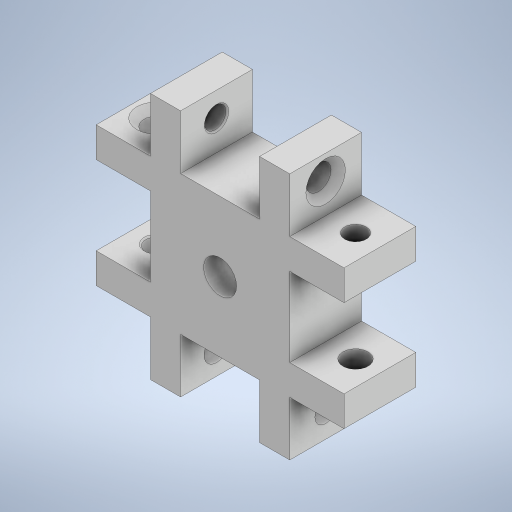
# Autodesk Inventor part: GripperMotorHinges
Saved by Autodesk Inventor 2023 (Build 270158000, 158)
## iProperties
Created: 2023-06-03
Part Number: GripperMotorHinges
Material: Ogólny
Document SubType Name: Modeling
Designer: Kamil
Density: 1 g/cm^3
Appearance: Domyślna
Author: Kamil
Autodesk Inventor part; units mm, degrees
ref_plane "YZ Plane" through (0, 0, 0) normal (1, 0, 0) x (0, 1, 0)
ref_plane "XZ Plane" through (0, 0, 0) normal (0, 1, 0) x (-1, 0, 0)
ref_plane "XY Plane" through (0, 0, 0) normal (0, 0, 1) x (1, 0, 0)
sketch "Szkic1" plane through (0, 0, 0) normal (0, 0, 1) x (1, 0, 0)
  line L0 (0, -7.56) -> (0, 0)
  line L1 (0, 19.4) -> (0, 26.96)
  line L2 (-4.2, 4.2) -> (-11.76, 4.2)
  line L3 (-11.76, 15.2) -> (-4.2, 15.2)
  line L4 (15.2, 15.2) -> (22.76, 15.2)
  line L5 (15.2, 4.2) -> (22.76, 4.2)
  line L6 (-4.2, 26.96) -> (-4.2, 19.4)
  line L7 (-4.2, 19.4) -> (-11.76, 19.4)
  line L8 (-4.2, 15.2) -> (-4.2, 4.2)
  line L9 (-4.2, 0) -> (-4.2, -7.56)
  line L10 (-11.76, 0) -> (-4.2, 0)
  line L11 (15.2, -7.56) -> (11, -7.56)
  line L12 (0, -7.56) -> (-4.2, -7.56)
  line L13 (0, 0) -> (11, 0)
  line L14 (15.2, 0) -> (22.76, 0)
  line L15 (11, 26.96) -> (11, 19.4)
  line L16 (11, 0) -> (11, -7.56)
  line L17 (15.2, -7.56) -> (15.2, 0)
  line L18 (15.2, 4.2) -> (15.2, 15.2)
  line L19 (15.2, 19.4) -> (15.2, 26.96)
  line L20 (22.76, 19.4) -> (15.2, 19.4)
  line L21 (11, 19.4) -> (0, 19.4)
  line L22 (22.76, 19.4) -> (22.76, 15.2)
  line L23 (22.76, 4.2) -> (22.76, 0)
  line L24 (-4.2, 26.96) -> (0, 26.96)
  line L25 (11, 26.96) -> (15.2, 26.96)
  line L26 (-11.76, 0) -> (-11.76, 4.2)
  line L27 (-11.76, 15.2) -> (-11.76, 19.4)
  circle A0 centre (5.5, 9.7) radius 2.3
  dimension "d0" = 4.6
  constraints: 56 end point, 8 parallel, 8 perpendicular, 2 horizontal, 1 centre point, 1 coincident
  measures "d0" diameter of A0
extrude "Wyciągnięcie proste1" add sketch "Szkic1" along normal blind 10
sketch "Szkic2" plane through (-11.76, 19.4, 0) normal (0, 1, 0) x (1, 0, 0)
  line L0 (7.56, 0) -> (0, 0) projected
  line L1 (0, 0) -> (0, -10) projected
  line L2 (7.56, -10) -> (0, -10) projected
  line L3 (7.56, 0) -> (7.56, -10) projected
  line L4 (34.52, 0) -> (26.96, 0) projected
  line L5 (26.96, 0) -> (26.96, -10) projected
  line L6 (34.52, -10) -> (26.96, -10) projected
  line L7 (34.52, 0) -> (34.52, -10) projected
  line L8 (0, 0) -> (0, -10) projected
  line L9 (0, -5) -> (3.4, -5)
  line L10 (34.52, 0) -> (34.52, -10) projected
  line L11 (34.52, -5) -> (31.12, -5)
  circle A0 centre (3.4, -5) radius 1.75
  circle A1 centre (31.12, -5) radius 1.75
  point P0 (11.76, 0)
  dimension "d3" = 3.4
  dimension "d4" = 3.4
  dimension "d5" = 3.5
  dimension "d6" = 3.5
  constraints: 4 end point, 2 centre point, 2 coincident, 2 horizontal, 2 midpoint
  measures "d3" distance of L9.start L9.end
  measures "d4" distance of L11.start L11.end
  measures "d5" diameter of A0
  measures "d6" diameter of A1
extrude "Wyciągnięcie proste2" cut sketch "Szkic2" against normal through all contours A0 | A1
sketch "Szkic3" plane through (-4.2, -7.56, 0) normal (-1, 0, 0) x (0, 0, 1)
  line L0 (0, 7.56) -> (0, 0) projected
  line L1 (0, 0) -> (10, 0) projected
  line L2 (10, 7.56) -> (10, 0) projected
  line L3 (0, 7.56) -> (10, 7.56) projected
  line L4 (0, 34.52) -> (0, 26.96) projected
  line L5 (0, 26.96) -> (10, 26.96) projected
  line L6 (10, 34.52) -> (10, 26.96) projected
  line L7 (0, 34.52) -> (10, 34.52) projected
  line L8 (5, 0) -> (5, 3.4)
  line L9 (0, 34.52) -> (10, 34.52) projected
  line L10 (5, 34.52) -> (5, 31.12)
  circle A0 centre (5, 3.4) radius 1.75
  circle A1 centre (5, 31.12) radius 1.75
  point P0 (0, 7.56)
  dimension "d9" = 3.4
  dimension "d10" = 3.4
  dimension "d11" = 3.5
  dimension "d12" = 3.5
  constraints: 4 end point, 2 centre point, 2 coincident, 2 midpoint, 2 vertical
  measures "d9" distance of L8.start L8.end
  measures "d10" distance of L10.start L10.end
  measures "d11" diameter of A0
  measures "d12" diameter of A1
extrude "Wyciągnięcie proste3" cut sketch "Szkic3" against normal through all contours A0 | A1
chamfer "Faza2" distance 1 angle 45 4 edges at (-4.2, -4.16, 3.25) (17.61, 0, 5) (15.2, 23.56, 3.25) (-10.11, 19.4, 5)
sketch "Szkic8" plane through (15.2, -7.56, 0) normal (1, 0, 0) x (0, 0, -1)
  circle A0 centre (-5, 3.4) radius 1.75 projected
  circle A1 centre (-5, 3.4) radius 1.5
  point P0 (0, 7.56)
  dimension "d42" = 3
  constraints: 1 centre point, 1 coincident
  measures "d42" diameter of A1
extrude "Wyciągnięcie proste8" add sketch "Szkic8" against normal up to surface (4.2 mm away)
pattern_circular "Szyk kołowy3" count 4 over 360 about axis through (5.5, 9.7, 0) along (0, 0, 1) of "Wyciągnięcie proste8"
chamfer "Faza3" distance 0.2 angle 45 4 edges at (11, -4.16, 6.5) (-8.36, 4.2, 6.5) (0, 23.56, 6.5) (19.36, 15.2, 6.5)
